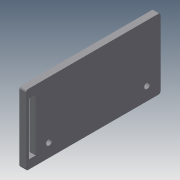
# Autodesk Inventor part: FrontLeft
Saved by Autodesk Inventor 2014 (Build 180170000, 170)
## iProperties
Created: 2015-02-17
Part Number: FrontLeft
Material: Generic
Document SubType Name: Modeling
Designer: Peele
Density: 1 g/cm^3
Appearance: Default
Author: Peele
Autodesk Inventor part; units mm, degrees
ref_plane "YZ Plane" through (0, 0, 0) normal (1, 0, 0) x (0, 1, 0)
ref_plane "XZ Plane" through (0, 0, 0) normal (0, 1, 0) x (-1, 0, 0)
ref_plane "XY Plane" through (0, 0, 0) normal (0, 0, 1) x (1, 0, 0)
sketch "Sketch1" plane through (0, 0, 0) normal (1, 0, 0) x (0, 1, 0)
  line L0 (0, 0) -> (125, 0)
  line L1 (125, 0) -> (125, 65)
  line L2 (125, 65) -> (0, 65)
  line L3 (0, 65) -> (0, 0)
  line L4 (2.875, 56.9) -> (9.125, 56.9)
  line L5 (9.125, 56.9) -> (9.125, 8.1)
  line L6 (9.125, 8.1) -> (2.875, 8.1)
  line L7 (2.875, 8.1) -> (2.875, 56.9)
  circle A0 centre (112.5, 12.5) radius 2.7
  circle A1 centre (21.5, 12.5) radius 2.7
  dimension "d0" = 65
  dimension "d1" = 125
  dimension "d2" = 6.25
  dimension "d3" = 2.875
  dimension "d4" = 8.1
  dimension "d5" = 8.1
  dimension "d6" = 12.5
  dimension "d7" = 21.5
  dimension "d8" = 12.5
  dimension "d9" = 5.4
  constraints: 16 end point, 4 parallel, 2 centre point, 2 horizontal, 2 perpendicular, 1 equal radius, 1 horizontal alignment
  measures "d0" distance of L2.end L0.start
  measures "d1" distance of L0.start L0.end
  measures "d2" distance of L4.start L4.end
  measures "d3" distance between parallel lines of L3 L7
  measures "d4" distance between parallel lines of L2 L4
  measures "d5" distance between parallel lines of L0 L6
  measures "d6" distance from line of A0.centre L1
  measures "d7" distance from line of L3 A1.centre
  measures "d8" distance from line of A0.centre L0
  measures "d9" diameter of A0
extrude "Extrusion1" add sketch "Sketch1" along normal blind 6
fillet "Fillet1" radius 2 4 edges at (3, 125, 65) (3, 125, 0) (3, 0, 65) (3, 0, 0)
equation "\"d5\" = d4"
body "Solid1"
